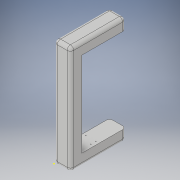
# Autodesk Inventor part: Bumper
Saved by Autodesk Inventor 2018 (Build 220112000, 112)
## iProperties
Created: 2018-01-19
Part Number: Bumper
Material: Generic
Document SubType Name: Modeling
Designer: s-4000369
Density: 1 g/cm^3
Appearance: Default
Author: s-4000369
Autodesk Inventor part; units mm, degrees
ref_plane "YZ Plane" through (0, 0, 0) normal (1, 0, 0) x (0, 1, 0)
ref_plane "XZ Plane" through (0, 0, 0) normal (0, 1, 0) x (-1, 0, 0)
ref_plane "XY Plane" through (0, 0, 0) normal (0, 0, 1) x (1, 0, 0)
sketch "Sketch1" plane through (0, 0, 0) normal (1, 0, 0) x (0, 1, 0)
  point P0 (0, 0)
sketch "Sketch2" plane through (0, 0, 0) normal (1, 0, 0) x (0, 1, 0)
  line L0 (0, 0) -> (0, -431.8)
  line L1 (0, -431.8) -> (88.9, -431.8)
  line L2 (88.9, -431.8) -> (88.9, -88.9)
  line L3 (88.9, -88.9) -> (749.3, -88.9)
  line L4 (749.3, -88.9) -> (749.3, -431.8)
  line L5 (749.3, -431.8) -> (838.2, -431.8)
  line L6 (838.2, -431.8) -> (838.2, 0)
  line L7 (838.2, 0) -> (0, 0)
  dimension "d0" = 660.4
  dimension "d1" = 342.9
  dimension "d2" = 342.9
  dimension "d3" = 88.9
  dimension "d4" = 88.9
  dimension "d5" = 88.9
  constraints: 16 end point, 6 perpendicular, 2 vertical
  measures "d0" distance of L2.end L3.end
  measures "d1" distance of L1.end L2.end
  measures "d2" distance of L3.end L4.end
  measures "d3" distance between parallel lines of L7 L3
  measures "d4" distance between parallel lines of L0 L2
  measures "d5" distance between parallel lines of L4 L6
extrude "Extrusion1" add sketch "Sketch2" along normal blind 127
fillet "Fillet1" radius 25.4 14 edges at (127, 419.1, 0) (0, 419.1, 0) (63.5, 838.2, 0) (127, 838.2, -215.9) (0, 838.2, -215.9) (63.5, 0, 0) (127, 0, -215.9) (127, 44.45, -431.8) (127, 793.75, -431.8) (63.5, 838.2, -431.8) (0, 793.75, -431.8) (0, 0, -215.9) (0, 44.45, -431.8) (63.5, 0, -431.8)
sketch "Sketch3" plane through (0, 88.9, -88.9) normal (0, 0, -1) x (-1, 0, 0)
  line L0 (0, 0) -> (-127, 0) projected
  line L1 (-63.5, 0) -> (-63.5, 660.4)
  line L2 (-25.4, 660.4) -> (-101.6, 660.4) projected
  line L3 (-63.5, 0) -> (-63.5, 254)
  line L4 (-63.5, 254) -> (-63.5, 406.4)
  line L5 (-63.5, 406.4) -> (-63.5, 660.4)
  line L6 (-63.5, 254) -> (-63.5, 292.1)
  line L7 (-63.5, 406.4) -> (-63.5, 368.3)
  circle A0 centre (-63.5, 292.1) radius 2.54
  circle A1 centre (-63.5, 368.3) radius 2.54
  line L8 (0, 0) -> (0, 660.4) projected
  line L9 (0, 406.4) -> (0, 368.3)
  line L10 (-127, 0) -> (-127, 660.4) projected
  line L11 (-60.96, 292.1) -> (-66.04, 292.1)
  line L12 (-63.5, 254) -> (-127, 254)
  line L13 (-127, 254) -> (-127, 292.1)
  line L14 (-127, 292.1) -> (-88.9, 292.1)
  line L15 (-127, 368.3) -> (-88.9, 368.3)
  line L16 (0, 292.1) -> (-38.1, 292.1)
  line L17 (0, 368.3) -> (-38.1, 368.3)
  circle A2 centre (-88.9, 292.1) radius 2.54
  circle A3 centre (-88.9, 368.3) radius 2.54
  circle A4 centre (-38.1, 368.3) radius 2.54
  circle A5 centre (-38.1, 292.1) radius 2.54
  point P0 (0, -88.9)
  dimension "d9" = 254
  dimension "d10" = 152.4
  dimension "d23" = 38.1
  dimension "d24" = 38.1
  dimension "d25" = 38.1
  constraints: 28 end point, 10 point on line, 6 centre point, 6 coincident, 4 horizontal, 3 perpendicular, 2 midpoint, 2 point on circle
  measures "d9" distance of L1.start L3.end
  measures "d10" distance of L3.end L4.end
  measures "d23" distance of L13.end L14.end
  measures "d24" distance of L9.end L17.end
  measures "d25" distance of L16.start L16.end
extrude "Extrusion2" cut sketch "Sketch3" against normal blind 3.175 contours A1 L1 | L1 A1 | A0 L11 L1 | L1 L11 A0 | L11 A0 L1 | L1 A0 L11
sketch "Sketch4" plane through (0, 88.9, -88.9) normal (0, 0, -1) x (-1, 0, 0)
  line L0 (0, 0) -> (-127, 0) projected
  line L1 (0, 0) -> (0, 292.1)
  line L2 (0, 0) -> (0, 660.4) projected
  line L3 (0, 292.1) -> (0, 368.3)
  line L4 (0, 292.1) -> (-38.1, 292.1)
  line L5 (0, 368.3) -> (-38.1, 368.3)
  line L6 (-127, 0) -> (-127, 660.4) projected
  line L7 (-127, 292.1) -> (-88.9, 292.1)
  line L8 (-127, 368.3) -> (-88.9, 368.3)
  circle A0 centre (-88.9, 292.1) radius 2.54
  circle A1 centre (-38.1, 292.1) radius 2.54
  circle A2 centre (-38.1, 368.3) radius 2.54
  circle A3 centre (-88.9, 368.3) radius 2.54
  point P0 (0, -88.9)
  dimension "d26" = 292.1
  dimension "d27" = 76.2
  dimension "d28" = 38.1
  dimension "d30" = 38.1
  dimension "d31" = 5.08
  dimension "d50" = 38.1
  dimension "d51" = 38.1
  constraints: 12 end point, 4 centre point, 4 coincident, 4 point on line, 2 horizontal, 2 perpendicular
  measures "d26" distance of L0.start L1.end
  measures "d27" distance of L1.end L3.end
  measures "d28" distance of L1.end L4.end
  measures "d30" distance of L7.start L7.end
  measures "d31" diameter of A0
  measures "d50" distance of L8.start L8.end
  measures "d51" distance of L3.end L5.end
extrude "Extrusion3" cut sketch "Sketch4" against normal blind 3.175
sketch "Sketch5" plane through (0, 749.3, -88.9) normal (0, -1, 0) x (1, 0, 0)
  line L0 (0, 0) -> (0, -317.5) projected
  line L1 (0, -152.3238) -> (87.3252, -152.3238)
  line L2 (25.4, -342.9) -> (101.6, -342.9) projected
  line L3 (127, 0) -> (127, -317.5) projected
  line L4 (127, -152.3238) -> (39.6748, -152.3238)
  circle A0 centre (87.3252, -152.3238) radius 2.54
  circle A1 centre (39.6748, -152.3238) radius 2.54
  line L5 (87.3252, -152.3238) -> (87.3252, -101.5238)
  line L6 (39.6748, -152.3238) -> (39.6748, -101.5238)
  circle A2 centre (39.6748, -101.5238) radius 2.54
  circle A3 centre (87.3252, -101.5238) radius 2.54
  line L7 (87.3252, -101.5238) -> (87.3252, 0)
  point P0 (0, 88.9)
  dimension "d34" = 87.3252
  dimension "d36" = 87.3252
  dimension "d37" = 5.08
  dimension "d40" = 50.8
  constraints: 10 end point, 4 centre point, 4 coincident, 3 point on line, 3 vertical, 1 horizontal
  measures "d34" distance of L1.start L1.end
  measures "d36" distance of L4.start L4.end
  measures "d37" diameter of A0
  measures "d40" distance of L5.start L5.end
extrude "Extrusion5" cut sketch "Sketch5" against normal blind 3.175
sketch "Sketch6" plane through (0, 88.9, -88.9) normal (0, 1, 0) x (1, 0, 0)
  arc A0 (127, 317.5) -> (101.6, 342.9) centre (101.6, 317.5) ccw projected
  line L0 (127, 317.5) -> (127, 0) projected
  line L1 (101.6, 317.5) -> (25.4, 317.5) projected
  line L2 (101.6, 317.5) -> (127, 317.5)
  line L3 (101.6, -63.5) -> (101.6, 317.5) projected
  line L4 (101.6, 317.5) -> (101.6, 133.35)
  line L5 (101.6, 133.35) -> (101.6, 95.25)
  line L6 (25.4, 133.35) -> (25.4, 95.25)
  circle A1 centre (101.6, 133.35) radius 2.54
  circle A2 centre (101.6, 95.25) radius 2.54
  circle A3 centre (25.4, 95.25) radius 2.54
  circle A4 centre (25.4, 133.35) radius 2.54
  line L7 (101.6, -88.9) -> (25.4, -88.9) projected
  line L8 (101.6, 317.5) -> (101.6, -88.9)
  line L9 (25.4, 95.25) -> (25.4, 0)
  point P0 (0, -88.9)
  dimension "d46" = 38.1
  dimension "d47" = 5.08
  constraints: 12 end point, 4 centre point, 4 coincident, 2 perpendicular, 2 point on line, 1 vertical
  measures "d46" distance of L4.end L5.end
  measures "d47" diameter of A1
extrude "Extrusion6" cut sketch "Sketch6" against normal blind 3.175
body "Solid1"
